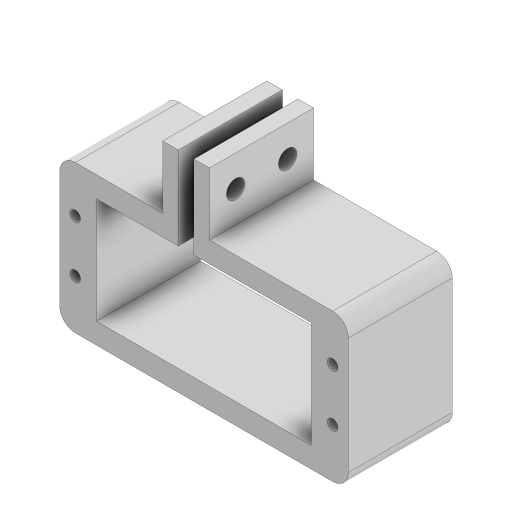
# Autodesk Inventor part: Servo mount
Saved by Autodesk Inventor 2024 (Build 280153000, 153)
## iProperties
Created: 2025-04-26
Part Number: Servo mount
Material: Generic
Document SubType Name: Modeling
Designer: Binara
Density: 1 g/cm^3
Appearance: Default
Author: Binara
Autodesk Inventor part; units mm, degrees
ref_plane "YZ Plane" through (0, 0, 0) normal (1, 0, 0) x (0, 1, 0)
ref_plane "XZ Plane" through (0, 0, 0) normal (0, 1, 0) x (-1, 0, 0)
ref_plane "XY Plane" through (0, 0, 0) normal (0, 0, 1) x (1, 0, 0)
sketch "Block1" plane through (0, 0, 0) normal (0, 0, 1) x (1, 0, 0)
  line L0 (-1.8704, 39.5395) -> (-1.8704, -10.4605)
  line L1 (-4.8704, 39.5395) -> (-4.8704, -10.4605)
  arc A0 (25.8721, -18.7556) -> (25.8721, -22.1655) centre (24.8076, -20.4605) ccw
  arc A1 (25.8721, -28.7556) -> (25.8721, -32.1655) centre (24.8076, -30.4605) ccw
  arc A2 (-25.7569, -32.1655) -> (-25.7569, -28.7556) centre (-24.6924, -30.4605) ccw
  arc A3 (-25.7569, -22.1655) -> (-25.7569, -18.7556) centre (-24.6924, -20.4605) ccw
  line L2 (10.765, -35.4505) -> (20.1076, -35.4505)
  line L3 (20.2076, -15.5605) -> (20.2076, -35.3605)
  line L4 (-20.0924, -15.5605) -> (-20.0924, -35.3605)
  point P0 (0.9099, -18.4595)
sketch "Sketch1" plane through (0, 0, 0) normal (0, 0, 1) x (1, 0, 0)
  circle A0 centre (24.8076, -18.2882) radius 1
  circle A1 centre (24.8076, -28.2882) radius 1
  circle A2 centre (-24.6924, -28.2882) radius 1
  circle A3 centre (-24.6924, -18.2882) radius 1
  line L0 (20.7076, -13.3882) -> (-20.5924, -13.3882)
  line L1 (-20.5924, -13.3882) -> (-20.5924, -33.7782)
  line L2 (-20.5924, -33.7782) -> (20.7076, -33.7782)
  line L3 (20.7076, -33.7782) -> (20.7076, -13.3882)
  line L4 (27.8076, -37.7782) -> (-27.6924, -37.7782)
  line L5 (-27.6924, -37.7782) -> (-27.6924, 2.6118)
  line L6 (-27.6924, 2.6118) -> (27.8076, 2.6118)
  line L7 (27.8076, 2.6118) -> (27.8076, -37.7782)
  line L8 (-1.8704, -8.2882) -> (-1.8704, -13.3882)
  line L9 (-4.8704, -8.2882) -> (-4.8704, -13.3882)
  line L10 (-27.6924, 2.6118) -> (-7.8704, 2.6118)
  line L11 (-7.8704, 2.6118) -> (-7.8704, -9.3882)
  line L12 (-7.8704, -9.3882) -> (-27.6924, -9.3882)
  line L13 (-27.6924, -9.3882) -> (-27.6924, 2.6118)
  line L14 (27.8076, 2.6118) -> (1.1296, 2.6118)
  line L15 (1.1296, 2.6118) -> (1.1296, -9.3882)
  line L16 (1.1296, -9.3882) -> (27.8076, -9.3882)
  line L17 (27.8076, -9.3882) -> (27.8076, 2.6118)
  line L18 (-1.8704, 41.7118) -> (-1.8704, -8.2882)
  line L19 (-4.8704, 41.7118) -> (-4.8704, -8.2882)
  arc A4 (25.8721, -16.5832) -> (25.8721, -19.9932) centre (24.8076, -18.2882) ccw
  arc A5 (25.8721, -26.5832) -> (25.8721, -29.9932) centre (24.8076, -28.2882) ccw
  arc A6 (-25.7569, -29.9932) -> (-25.7569, -26.5832) centre (-24.6924, -28.2882) ccw
  arc A7 (-25.7569, -19.9932) -> (-25.7569, -16.5832) centre (-24.6924, -18.2882) ccw
  line L20 (10.765, -33.2782) -> (20.1076, -33.2782)
  line L21 (20.2076, -13.3882) -> (20.2076, -33.1882)
  line L22 (-20.0924, -13.3882) -> (-20.0924, -33.1882)
  point P0 (0, 0)
  point P1 (15.4363, -33.2782)
  point P2 (-4.8704, -8.2882)
  point P3 (-4.8704, 2.6118)
  point P4 (-1.8704, 2.6118)
  point P5 (-1.8704, -8.2882)
  dimension "d0" = 2
  dimension "d1" = 2
  dimension "d2" = 2
  dimension "d3" = 2
  dimension "d4" = 0.5
  dimension "d5" = 0.5
  dimension "d6" = 0.5
  dimension "d7" = 3
  dimension "d8" = 3
  dimension "d9" = 3
  dimension "d10" = 3
  dimension "d11" = 12
  dimension "d12" = 12
  dimension "d13" = 4
  dimension "d14" = 4
  constraints: 36 end point, 8 parallel, 5 horizontal, 5 perpendicular, 4 centre point, 2 point on line, 1 vertical, 7 other
  measures "d0" diameter of A0
  measures "d1" diameter of A1
  measures "d2" diameter of A2
  measures "d3" diameter of A3
  measures "d5" distance from line of L2 point (15.436, -33.278)
  measures "d11" distance of L14.end L15.end
  measures "d12" distance of L10.end L11.end
  measures "d13" distance between parallel lines of L0 L16
  measures "d14" distance between parallel lines of L2 L4
extrude "Extrusion1" add sketch "Sketch1" along normal blind 20 contours L0 L8 L18 L6 L15 L16 L7 L4 L5 L12 L11 L19 L9 L1 L2 L3
sketch "Sketch2" plane through (-7.8704, -9.3882, 0) normal (-1, 0, 0) x (0, 0, 1)
  line L0 (0, 12) -> (0, 0) projected
  line L1 (0, 0) -> (20, 0) projected
  line L2 (20, 12) -> (20, 0) projected
  line L3 (0, 12) -> (20, 12) projected
  line L4 (20, 6) -> (0, 6)
  line L5 (0, -4) -> (0, 12) projected
  circle A0 centre (15, 6) radius 1.75
  circle A1 centre (5, 6) radius 1.75
  point P0 (0, 9.3882)
  dimension "d17" = 3.5
  dimension "d18" = 3.5
  dimension "d19" = 10
  dimension "d20" = 20
  dimension "d21" = 5
  constraints: 3 point on line, 2 centre point, 2 end point, 1 midpoint, 1 perpendicular
  measures "d17" diameter of A0
  measures "d18" diameter of A1
  measures "d19" distance of A1.centre A0.centre
  measures "d20" distance of L4.start L4.end
  measures "d21" distance from line of L2 A0.centre
extrude "Extrusion2" cut sketch "Sketch2" against normal blind 20 contours A1 L4 | L4 A1 | A0 L4 | L4 A0
fillet "Fillet1" radius 3 4 edges at (27.8076, -9.3882, 10) (27.8076, -37.7782, 10) (-27.6924, -37.7782, 10) (-27.6924, -9.3882, 10)
equation "\"d6\" = d4"
equation "\"d12\" = d11"
body "Solid1"
